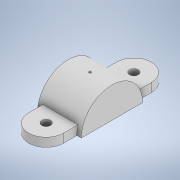
# Autodesk Inventor part: ch7-parent
Saved by Autodesk Inventor 2020 (Build 240168000, 168)
## iProperties
Created: 2020-02-28
Part Number: ch7-parent
Material: Generic
Document SubType Name: Modeling
Designer: Eric
Density: 1 g/cm^3
Appearance: Default
Author: Eric
Autodesk Inventor part; units mm, degrees
ref_plane "YZ Plane" through (0, 0, 0) normal (1, 0, 0) x (0, 1, 0)
ref_plane "XZ Plane" through (0, 0, 0) normal (0, 1, 0) x (-1, 0, 0)
ref_plane "XY Plane" through (0, 0, 0) normal (0, 0, 1) x (1, 0, 0)
sketch "Sketch1" plane through (0, 0, 0) normal (0, 1, 0) x (-1, 0, 0)
  line L0 (0, 63.5) -> (0, -63.5) construction
  line L1 (-25.4, 63.5) -> (-25.4, -63.5)
  line L2 (25.4, -63.5) -> (25.4, 63.5)
  arc A0 (25.4, 63.5) -> (-25.4, 63.5) centre (0, 63.5) ccw
  arc A1 (-25.4, -63.5) -> (25.4, -63.5) centre (0, -63.5) ccw
  circle A2 centre (0, 63.5) radius 6.35
  circle A3 centre (0, -63.5) radius 6.35
  point P0 (0, 0)
  dimension "d0" = 127
  dimension "d1" = 25.4
  dimension "d2" = 12.7
  constraints: 8 end point, 4 centre point, 4 point on circle, 4 tangent, 2 coincident, 1 equal radius, 1 midpoint, 1 parallel, 1 vertical
  measures "d0" distance of L0.end L0.start
  measures "d1" radius of A1
  measures "d2" diameter of A3
extrude "Extrusion1" add sketch "Sketch1" along normal blind 12.7
sketch "Sketch2" plane through (0, 0, 0) normal (1, 0, 0) x (0, 1, 0)
  arc A0 (0, -44.45) -> (0, 44.45) centre (0, 0) ccw
  line L0 (0, 44.45) -> (0, -44.45)
  line L1 (0, 63.5) -> (0, -63.5) projected
  dimension "d5" = 44.45
  constraints: 2 end point, 2 point on circle, 1 centre point, 1 coincident, 1 collinear, 1 vertical
  measures "d5" radius of A0
extrude "Extrusion2" add sketch "Sketch2" along normal mid plane 63.5
sketch "Sketch3" plane through (31.75, 0, 0) normal (1, 0, 0) x (0, 0, -1)
  line L0 (-25.4, 0) -> (25.4, 0)
  line L1 (25.4, 0) -> (25.4, 19.05)
  line L2 (25.4, 19.05) -> (-25.4, 19.05)
  line L3 (-25.4, 19.05) -> (-25.4, 0)
  point P0 (0, 0)
  point P1 (0, 19.05)
  point P2 (0, 0)
  dimension "d8" = 50.8
  dimension "d9" = 19.05
  constraints: 8 end point, 2 midpoint, 2 parallel, 2 vertical alignment, 1 horizontal, 1 horizontal alignment, 1 perpendicular
  measures "d8" distance of L1.end L2.end
  measures "d9" distance of L2.end L0.start
extrude "rectCut" [suppressed]
sketch "Sketch4" plane through (31.75, 0, -25.4) normal (0, -1, 0) x (1, 0, 0)
  circle A0 centre (-31.75, 25.4) radius 1.5875
  dimension "d12" = 3.175
  constraints: 1 centre point, 1 coincident
  measures "d12" diameter of A0
extrude ".125Hole" cut sketch "Sketch4" against normal through all
sketch "Sketch5" plane through (31.75, 0, 0) normal (1, 0, 0) x (0, 0, -1)
  arc A0 (31.75, 0) -> (-31.75, 0) centre (0, 0) ccw
  line L0 (31.75, 0) -> (-31.75, 0)
  dimension "d15" = 31.75
  constraints: 2 end point, 2 point on circle, 1 centre point, 1 coincident, 1 horizontal, 1 horizontal alignment
  measures "d15" radius of A0
extrude "circCut" [suppressed]
body "Solid1"
